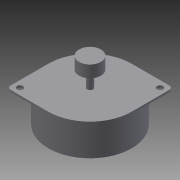
# Autodesk Inventor part: stepper motor 1
Saved by Autodesk Inventor 2013 (Build 170138000, 138)
## iProperties
Created: 2017-01-29
Part Number: stepper motor 1
Material: Generic
Document SubType Name: Modeling
Designer: Herman de Vries
Density: 1 g/cm^3
Author: Herman de Vries
Autodesk Inventor part; units mm, degrees
ref_plane "YZ Plane" through (0, 0, 0) normal (1, 0, 0) x (0, 1, 0)
ref_plane "XZ Plane" through (0, 0, 0) normal (0, 1, 0) x (-1, 0, 0)
ref_plane "XY Plane" through (0, 0, 0) normal (0, 0, 1) x (1, 0, 0)
sketch "Sketch1" plane through (0, 0, 0) normal (0, 0, 1) x (1, 0, 0)
  circle A0 centre (0, 0) radius 21
  dimension "d0" = 42
  constraints: 1 centre point, 1 coincident
  measures "d0" diameter of A0
extrude "Extrusion1" add sketch "Sketch1" along normal blind 15
sketch "Sketch2" plane through (0, 0, 15) normal (0, 0, 1) x (1, 0, 0)
  circle A0 centre (0, 0) radius 21 construction
  circle A1 centre (0, 0) radius 1.5
  dimension "d3" = 3
  constraints: 1 centre point, 1 coincident
  measures "d3" diameter of A1
extrude "Extrusion2" add sketch "Sketch2" along normal blind 15
sketch "Sketch3" plane through (0, 0, 15) normal (0, 0, 1) x (1, 0, 0)
  circle A0 centre (0, 0) radius 1.5 construction
  circle A1 centre (0, 0) radius 21 construction
  line L0 (-19, -21) -> (0, -21)
  line L1 (21, 0) -> (21, 19)
  line L2 (19, 21) -> (0, 21)
  line L3 (-21, 0) -> (-21, -19)
  line L4 (-21, -21) -> (21, 21) construction
  line L5 (21, -21) -> (-21, 21) construction
  circle A2 centre (0, 0) radius 21 projected
  arc A3 (21, 19) -> (19, 21) centre (19, 19) ccw
  arc A4 (-21, -19) -> (-19, -21) centre (-19, -19) ccw
  circle A5 centre (-17.6777, -17.6777) radius 1.5
  circle A6 centre (17.6777, 17.6777) radius 1.5
  point P0 (0, 0)
  dimension "d6" = 2
  dimension "d7" = 3
  dimension "d8" = 3
  dimension "d9" = 25
  dimension "d10" = 25
  constraints: 12 end point, 8 point on circle, 6 point on line, 6 tangent, 4 centre point, 3 midpoint, 2 parallel, 1 coincident, 1 equal radius, 1 horizontal, 1 perpendicular
  measures "d6" radius of A3
  measures "d7" diameter of A5
  measures "d8" diameter of A6
  measures "d9" distance of point (0, 0) A5.centre
  measures "d10" distance of point (0, 0) A6.centre
extrude "Extrusion3" add sketch "Sketch3" along normal blind 1
sketch "Sketch4" plane through (0, 0, 30) normal (0, 0, 1) x (1, 0, 0)
  circle A0 centre (0, 0) radius 5.5
  dimension "d13" = 11
  constraints: 1 centre point, 1 coincident
  measures "d13" diameter of A0
extrude "Extrusion4" add sketch "Sketch4" against normal blind 6
equation "\"d10\" = d9"
body "Solid1"
